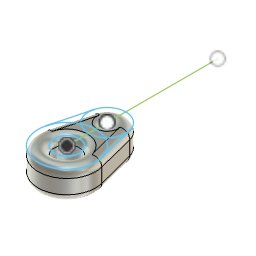
mmono (Autodesk Fusion 360 design; units mm, degrees)
Autodesk Fusion 360 part; units mm, degrees
sketch "Sketch1" plane through (0, 0, 0) normal (0, 0, 1) x (1, 0, 0)
  line L0 (0, -0.0218) -> (0, 150)
  circle A0 centre (0, -0.0218) radius 12.5
  circle A1 centre (0, -0.0218) radius 28.5
  circle A2 centre (0.0333, 39.9782) radius 2.5
  circle A3 centre (0.0333, 39.9782) radius 18.5
  line L1 (17.9497, 44.5882) -> (27.6009, 7.0802)
  line L2 (-17.8754, 44.6181) -> (-27.5891, 7.1262)
  dimension "d38" = 16
  dimension "d39" = 25
  dimension "d40" = 5
  dimension "d42" = 40
  dimension "d43" = 16
  constraint coincident L0.start A0.centre
  constraint coincident A3 L1.start
  constraint tangent A3 L1
  constraint coincident A1 L1.end
  constraint tangent A1 L1
  constraint coincident A3 L2.start
  constraint tangent A3 L2
  constraint coincident A1 L2.end
  constraint tangent A1 L2
  measures "d39" diameter of A0
  measures "d40" diameter of A2
  measures "d42" distance of L0.start A2.centre
extrude "Extrude6" add sketch "Sketch1" against normal blind 30 contours L0 A1 A3 | A1 A3 | L0 A1 A3 | L0 A1 A2 A3 | L0 A1 A2 A3 | A1 A3 L2 | A1 A3 L1 | A0
extrude "Extrude7" cut sketch "Sketch1" against normal blind 22.3431 contours A0
fillet "Fillet2" radius 8 1 edges at (-11.6541, 4.4984, 0)
fillet "Fillet2" radius 8 2 edges at (-2.2975, 40.8822, 0) (-2.2975, 39.0741, -30)
fillet "Fillet2" radius 8 8 edges at (-0.0237, -28.5218, 0) (22.7753, 25.8342, 0) (0.0487, 58.4782, 0) (-22.7322, 25.8721, 0) (-22.7322, 25.8721, -30) (0.0487, 58.4782, -30) (22.7753, 25.8342, -30) (-0.0237, -28.5218, -30)
